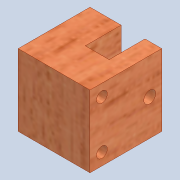
# Autodesk Inventor part: 0005-10-018 intinzator x
Saved by Autodesk Inventor 2020 (Build 240168000, 168)
## iProperties
Created: 2020-12-19
Part Number: 0005-10-018 intinzator x
Material: Wood (Maple)
Document SubType Name: Modeling
Designer: Iulian Bors
Density: 0.67 g/cm^3
Appearance: Red Oak - Natural Low Gloss
Mass: 14.2266 g
Surface Area: 69.9729 cm^2
Volume: 21.2338 cm^3
Author: Iulian Bors
Subject: 018
Autodesk Inventor part; units mm, degrees
ref_plane "YZ Plane" through (0, 0, 0) normal (1, 0, 0) x (0, 1, 0)
ref_plane "XZ Plane" through (0, 0, 0) normal (0, 1, 0) x (-1, 0, 0)
ref_plane "XY Plane" through (0, 0, 0) normal (0, 0, 1) x (1, 0, 0)
sketch "Sketch1" plane through (0, 0, 0) normal (0, 0, 1) x (1, 0, 0)
  line L0 (-15, 15) -> (15, 15)
  line L1 (15, 15) -> (15, -15)
  line L2 (15, -15) -> (-15, -15)
  line L3 (-15, -15) -> (-15, 15)
  point P0 (0, 0)
  point P1 (0, 15)
  point P2 (-15, 0)
  dimension "d0" = 30
  dimension "d1" = 30
  constraints: 8 end point, 2 midpoint, 2 parallel, 1 horizontal, 1 horizontal alignment, 1 perpendicular, 1 vertical alignment
  measures "d0" distance of L0.start L0.end
  measures "d1" distance of L0.end L1.end
extrude "Extrusion1" add sketch "Sketch1" along normal blind 30
sketch "Sketch6" plane through (15, -15, 0) normal (1, 0, 0) x (0, 0, -1)
  circle A0 centre (-25, 5) radius 2.25
  circle A1 centre (-25, 25) radius 2.25
  line L0 (-30, 0) -> (-30, 30) projected
  line L1 (0, 0) -> (-30, 0) projected
  line L2 (0, 30) -> (-30, 30) projected
  point P0 (0, 15)
  dimension "d19" = 4.5
  dimension "d20" = 5
  dimension "d21" = 5
  dimension "d22" = 5
  constraints: 2 centre point, 1 equal radius, 1 vertical alignment
  measures "d19" diameter of A1
  measures "d20" distance from line of A0.centre L0
  measures "d21" distance from line of A0.centre L1
  measures "d22" distance from line of L2 A1.centre
extrude "Extrusion4" cut sketch "Sketch6" against normal through all
sketch "Sketch4" plane through (0, 0, 0) normal (0, 0, -1) x (-1, 0, 0)
  line L0 (2, -15) -> (-8, -15)
  line L1 (-8, -15) -> (-8, 15)
  line L2 (-8, 15) -> (2, 15)
  line L3 (2, 15) -> (2, -15)
  line L4 (15, -15) -> (-15, -15) projected
  line L5 (-15, 15) -> (15, 15) projected
  line L6 (-15, -15) -> (-15, 15) projected
  point P0 (0, 0)
  dimension "d8" = 10
  dimension "d25" = 7
  constraints: 8 end point, 2 collinear, 2 parallel, 1 horizontal, 1 perpendicular
  measures "d8" distance of L0.start L0.end
  measures "d25" distance between parallel lines of L6 L1
extrude "Extrusion3" cut sketch "Sketch4" against normal blind 15 contours L0 L1 L2 L3
sketch "Sketch5" plane through (15, -15, 0) normal (1, 0, 0) x (0, 0, -1)
  line L0 (0, 0) -> (0, 30) projected
  point P0 (0, 15)
  point P1 (-5, 15)
  point P2 (0, 15)
  dimension "d11" = 5
  constraints: 1 horizontal alignment, 1 midpoint
  measures "d11" distance of point (0, 15) point (-5, 15)
hole "Hole1" at (15, 0, 5) direction (-1, 0, 0) diameter 5 depth 10 tip angle 118
sketch "Sketch7" plane through (-2, -15, 0) normal (1, 0, 0) x (0, 0, -1)
  circle A0 centre (-5, 15) radius 2.5 projected
  point P0 (0, 15)
  constraints: 1 coincident
hole "Hole2" at (-2, 0, 5) direction (-1, 0, 0) diameter 4.134 end through all thread size "M5x0.8" class "6H" standard "ISO Metric profile"
equation "\"d22\" = d21"
body "Solid1"
